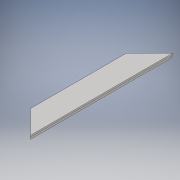
# Autodesk Inventor part: Upper Base Plate
Saved by Autodesk Inventor 2019.1 (Build 231200000, 200)
## iProperties
Created: 2020-12-23
Part Number: Upper Base Plate
Material: Generic
Document SubType Name: Modeling
Designer: Thomas Dodd
Density: 1 g/cm^3
Appearance: Default
Author: Thomas Dodd
Autodesk Inventor part; units mm, degrees
ref_plane "YZ Plane" through (0, 0, 0) normal (1, 0, 0) x (0, 1, 0)
ref_plane "XZ Plane" through (0, 0, 0) normal (0, 1, 0) x (-1, 0, 0)
ref_plane "XY Plane" through (0, 0, 0) normal (0, 0, 1) x (1, 0, 0)
sketch "Sketch1" plane through (0, 0, 0) normal (0, 1, 0) x (-1, 0, 0)
  line L0 (0, 0) -> (0, -5) construction
  line L1 (0, -5) -> (17, -5) construction
  line L2 (17, -5) -> (27, -5)
  line L3 (17, -5) -> (17, 0) construction
  line L4 (17, 0) -> (0, 0) construction
  spline S0 degree 2 poles (17, -5) (17, 0) (0, 0) knots 1 1 1 2 2 2
  line L5 (17, 0) -> (17, -5)
  line L6 (27, -5) -> (27, 0)
  line L7 (27, 0) -> (27, 140)
  line L8 (27, 140) -> (0, 140)
  line L9 (0, 140) -> (0, 0)
  dimension "d0" = 5
  dimension "d1" = 17
  dimension "d2" = 10
  dimension "d5" = 5
  dimension "d6" = 140
  dimension "d7" = 145
  constraints: 16 end point, 4 perpendicular, 3 vertical, 1 coincident, 1 point on line, 3 other
  measures "d0" distance of L0.start L0.end
  measures "d1" distance of L0.end L1.end
  measures "d2" distance of L1.end L2.end
  measures "d5" distance from line of L2 L3.end
  measures "d6" distance of L6.end L7.end
  measures "d7" distance between parallel lines of L8 L2
extrude "Extrusion1" add sketch "Sketch1" along normal blind 890
sketch "Sketch2" plane through (-27, 0, -5) normal (-1, 0, 0) x (0, 0, 1)
  line L0 (145, 0) -> (145, 890) projected
  line L1 (0, 0) -> (145, 0) projected
  line L2 (0, 0) -> (145, 145)
  line L3 (0, 0) -> (205.061, 0) construction
  line L4 (0, 890) -> (145, 890) projected
  line L5 (0, 890) -> (145, 745)
  line L6 (0, 890) -> (205.061, 890) construction
  point P0 (5, 0)
  dimension "d10" = 45
  dimension "d11" = 45
  constraints: 8 end point, 2 equal length, 2 horizontal, 2 point on line
  measures "d10" angle of L3 L2
  measures "d11" angle of L5 L6
extrude "Extrusion2" cut sketch "Sketch2" against normal blind 885
body "Solid1"
